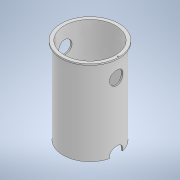
# Autodesk Inventor part: Втулка
Saved by Autodesk Inventor 2021 (Build 250183000, 183)
## iProperties
Created: 2020-11-11
Part Number: Втулка
Material: Типовые
Document SubType Name: Modeling
Designer: Тимоха
Density: 1 g/cm^3
Appearance: По умолчанию
Author: Тимоха
Autodesk Inventor part; units mm, degrees
ref_plane "YZ Plane" through (0, 0, 0) normal (1, 0, 0) x (0, 1, 0)
ref_plane "XZ Plane" through (0, 0, 0) normal (0, 1, 0) x (-1, 0, 0)
ref_plane "XY Plane" through (0, 0, 0) normal (0, 0, 1) x (1, 0, 0)
sketch "Эскиз1" plane through (0, 0, 0) normal (0, 0, 1) x (1, 0, 0)
  line L0 (0, 0) -> (190, 0)
  line L1 (190, 0) -> (190, 640)
  line L2 (190, 640) -> (215, 640)
  line L3 (215, 640) -> (215, 630)
  line L4 (215, 630) -> (200, 630)
  line L5 (200, 630) -> (200, 0)
  line L6 (200, 0) -> (190, 0)
  line L7 (0, -128) -> (0, 768) projected
  dimension "d0" = 190
  dimension "d1" = 640
  dimension "d2" = 25
  dimension "d3" = 10
  constraints: 14 end point, 5 perpendicular, 1 horizontal, 1 vertical
  measures "d0" distance of L0.start L0.end
  measures "d1" distance of L0.end L1.end
  measures "d2" distance of L1.end L2.end
  measures "d3" distance of L2.end L3.end
revolve "Вращение1" add sketch "Эскиз1" angle 360 about axis through (0, -10, 0) along (0, 1, 0)
sketch "Эскиз2" plane through (0, 640, 0) normal (0, 1, 0) x (1, 0, 0)
  circle A0 centre (207.2834, 0) radius 4
  point P0 (0, 0)
  dimension "d6" = 8
  constraints: 1 centre point
  measures "d6" diameter of A0
extrude "Выдавливание1" cut sketch "Эскиз2" against normal through all
sketch "Эскиз3" plane through (0, 0, 0) normal (1, 0, 0) x (0, 1, 0)
  line L0 (630, 215) -> (630, -215) projected
  line L1 (630, 200) -> (630, -200) projected
  line L2 (630, 0) -> (499, 0)
  circle A0 centre (499, 0) radius 50
  line L3 (0, 0) -> (11.003, 0)
  circle A1 centre (11.003, 0) radius 50
  dimension "d11" = 131
  dimension "d12" = 100
  dimension "d17" = 11.003
  dimension "d18" = 100
  constraints: 4 end point, 2 centre point, 2 coincident, 2 horizontal, 1 midpoint
  measures "d11" distance of L2.start L2.end
  measures "d12" diameter of A0
  measures "d17" distance of L3.start L3.end
  measures "d18" diameter of A1
extrude "Выдавливание2" cut sketch "Эскиз3" along normal through all both and the other way through all
